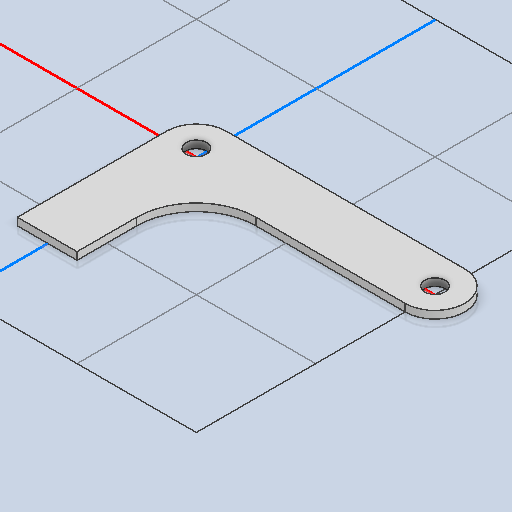
# Autodesk Inventor part: Magazine Gusset
Saved by Autodesk Inventor 2026 (Build 300175000, 175)
## iProperties
Created: 2025-04-07
Part Number: Magazine Gusset
Material: Generic
Document SubType Name: Modeling
Designer: avere
Density: 1 g/cm^3
Appearance: Default
d0: 0.500 in
d1: 0.500 in
d2: 0.500 in
d5: 2.000 in
d6: 0.500 in
Author: avere
Autodesk Inventor part; units mm, degrees
ref_plane "YZ Plane" through (0, 0, 0) normal (1, 0, 0) x (0, 1, 0)
ref_plane "XZ Plane" through (0, 0, 0) normal (0, 1, 0) x (-1, 0, 0)
ref_plane "XY Plane" through (0, 0, 0) normal (0, 0, 1) x (1, 0, 0)
sketch "main" plane through (0, 0, 0) normal (0, 0, 1) x (1, 0, 0)
  circle A0 centre (13.5257, -15.1463) radius 2.1844
  circle A1 centre (-37.2743, -15.1463) radius 2.1844
  arc A2 (13.5257, -21.4963) -> (19.8757, -15.1463) centre (13.5257, -15.1463) ccw
  arc A3 (-37.2743, -8.7963) -> (-37.2743, -21.4963) centre (-37.2743, -15.1463) ccw
  line L0 (7.1757, 10.2537) -> (7.1757, 3.9037)
  line L1 (-5.5243, -8.7963) -> (-37.2743, -8.7963)
  arc A4 (-5.5243, -8.7963) -> (7.1757, 3.9037) centre (-5.5243, 3.9037) ccw
  line L2 (19.8757, 16.6037) -> (19.8757, -15.1463)
  line L3 (13.5257, -21.4963) -> (-37.2743, -21.4963)
  line L4 (7.1757, 10.2537) -> (7.1757, 16.6037)
  line L5 (7.1757, 16.6037) -> (19.8757, 16.6037)
  point P0 (6.3402, -4.1174)
  dimension "d0" = 12.7
  dimension "d1" = 12.7
  dimension "d2" = 12.7
  dimension "d5" = 50.8
  dimension "d6" = 12.7
  measures "d0" diameter of A2
  measures "d1" diameter of A3
  measures "d2" radius of A4
  measures "d5" distance of A2.centre A3.centre
  measures "d6" distance of L4.end L2.start
sketch "Sketch1" plane through (0, 0, 0) normal (0, 1, 0) x (-1, 0, 0)
  circle A0 centre (0, 0) radius 2.1844
  circle A1 centre (-50.8, 0) radius 2.1844
  arc A2 (0, -6.35) -> (6.35, 0) centre (0, 0) ccw
  arc A3 (-50.8, 6.35) -> (-50.8, -6.35) centre (-50.8, 0) ccw
  line L0 (-6.35, 25.4) -> (-6.35, 19.05)
  line L1 (-19.05, 6.35) -> (-50.8, 6.35)
  arc A4 (-19.05, 6.35) -> (-6.35, 19.05) centre (-19.05, 19.05) ccw
  line L2 (6.35, 31.75) -> (6.35, 0)
  line L3 (0, -6.35) -> (-50.8, -6.35)
  line L4 (-6.35, 25.4) -> (-6.35, 31.75)
  line L5 (-6.35, 31.75) -> (6.35, 31.75)
  constraints: 1 other
extrude "Extrusion1" add sketch "Sketch1" along normal blind 1.5875
body "Solid1"
